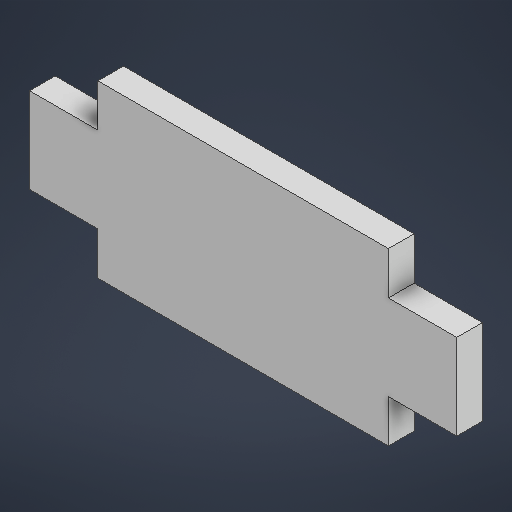
# Autodesk Inventor part: Frontrail
Saved by Autodesk Inventor 2027 (Build 310192000, 192)
## iProperties
Created: 2026-05-13
Part Number: Frontrail
Material: Generic
Document SubType Name: Modeling
Designer: alexy
Density: 1 g/cm^3
Appearance: Default
Author: alexy
Autodesk Inventor part; units mm, degrees
ref_plane "YZ Plane" through (0, 0, 0) normal (1, 0, 0) x (0, 1, 0)
ref_plane "XZ Plane" through (0, 0, 0) normal (0, 1, 0) x (-1, 0, 0)
ref_plane "XY Plane" through (0, 0, 0) normal (0, 0, 1) x (1, 0, 0)
sketch "Sketch1" plane through (0, 0, 0) normal (0, 0, 1) x (1, 0, 0)
  line L0 (0, 0) -> (34, 0)
  line L1 (34, 0) -> (34, 20)
  line L2 (34, 20) -> (0, 20)
  line L3 (0, 20) -> (0, 0)
  line L4 (-8, 15) -> (0, 15)
  line L5 (0, 15) -> (0, 5)
  line L6 (0, 5) -> (-8, 5)
  line L7 (-8, 5) -> (-8, 15)
  line L8 (-8, 15) -> (0, 5) construction
  line L9 (0, 15) -> (-8, 5) construction
  line L10 (42, 15) -> (34, 15)
  line L11 (34, 15) -> (34, 5)
  line L12 (34, 5) -> (42, 5)
  line L13 (42, 5) -> (42, 15)
  line L14 (42, 15) -> (34, 5) construction
  line L15 (34, 15) -> (42, 5) construction
  point P0 (-4, 10)
  point P1 (38, 10)
  point P2 (0, 10)
  point P3 (0, 10)
  point P4 (34, 15)
  point P5 (0, 15)
  dimension "d0" = 34
  dimension "d1" = 20
  dimension "d2" = 8
  dimension "d3" = 8
  dimension "d4" = 10
  dimension "d5" = 10
  constraints: 32 end point, 6 midpoint, 6 parallel, 3 horizontal, 3 perpendicular, 2 horizontal alignment, 2 point on line
  measures "d0" distance of L1.end L2.end
  measures "d1" distance of L0.end L1.end
  measures "d2" distance of L10.start L10.end
  measures "d3" distance of L4.start L4.end
  measures "d4" distance of L6.end L4.start
  measures "d5" distance of L12.end L10.start
extrude "Extrusion1" add sketch "Sketch1" along normal blind 3
body "Solid1"
